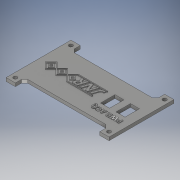
# Autodesk Inventor part: MapleMiniCase_TopCover
Saved by Autodesk Inventor 2018 (Build 220112000, 112)
## iProperties
Created: 2019-01-14
Part Number: MapleMiniCase_TopCover
Material: Generic
Document SubType Name: Modeling
Designer: tbrow
Density: 1 g/cm^3
Appearance: Default
Author: tbrow
## iProperties of the stored document MapleMiniCase_TopCover_3DPrint.ipt
Created: 2019-01-15
Part Number: MapleMiniCase_TopCover_3DPrint
Material: Generic
Document SubType Name: Modeling
Designer: tbrow
Density: 1 g/cm^3
Appearance: Default
Author: tbrow
Autodesk Inventor part; units mm, degrees
ref_plane "YZ Plane" through (0, 0, 0) normal (1, 0, 0) x (0, 1, 0)
ref_plane "XZ Plane" through (0, 0, 0) normal (0, 1, 0) x (-1, 0, 0)
ref_plane "XY Plane" through (0, 0, 0) normal (0, 0, 1) x (1, 0, 0)
sketch "Sketch1" plane through (0, 0, 0) normal (0, 1, 0) x (-1, 0, 0)
  line L0 (0, 0) -> (9.144, 0)
  line L1 (9.144, 0) -> (9.144, -9.144)
  line L2 (9.144, -9.144) -> (89.916, -9.144)
  line L3 (89.916, -9.144) -> (89.916, 0)
  line L4 (89.916, 0) -> (99.06, 0)
  line L5 (99.06, 0) -> (99.06, -58.6994)
  line L6 (99.06, -58.6994) -> (89.916, -58.6994)
  line L7 (89.916, -58.6994) -> (89.916, -49.5554)
  line L8 (89.916, -49.5554) -> (9.144, -49.5554)
  line L9 (9.144, -49.5554) -> (9.144, -58.6994)
  line L10 (9.144, -58.6994) -> (0, -58.6994)
  line L11 (0, -58.6994) -> (0, 0)
  dimension "d0" = 58.6994
  dimension "d1" = 9.144
  dimension "d2" = 9.144
  dimension "d3" = 9.144
  dimension "d4" = 9.144
  dimension "d5" = 9.144
  dimension "d7" = 9.144
  dimension "d16" = 99.06
  constraints: 24 end point, 8 perpendicular, 4 point on line, 2 horizontal
  measures "d0" distance of L4.end L5.end
  measures "d1" distance of L3.end L4.end
  measures "d2" distance of L2.end L3.end
  measures "d3" distance of L6.end L7.end
  measures "d4" distance of L0.start L0.end
  measures "d5" distance of L9.end L10.end
  measures "d7" distance of L5.end L6.end
  measures "d16" distance between parallel lines of L11 L5
extrude "Extrusion1" add sketch "Sketch1" along normal blind 3.175
sketch "Sketch2" plane through (0, 3.175, 0) normal (0, 1, 0) x (1, 0, 0)
  line L0 (-99.06, 0) -> (-89.916, 0) projected
  line L1 (-89.916, 58.6994) -> (-99.06, 58.6994) projected
  line L2 (-89.916, 49.5554) -> (-89.916, 58.6994) projected
  line L3 (-89.916, 0) -> (-89.916, 9.144) projected
  line L4 (-9.144, 0) -> (0, 0) projected
  line L5 (-9.144, 9.144) -> (-9.144, 0) projected
  line L6 (-9.144, 58.6994) -> (-9.144, 49.5554) projected
  circle A0 centre (-94.488, 4.572) radius 1.8542
  circle A1 centre (-94.488, 54.102) radius 1.8542
  circle A2 centre (-4.572, 54.102) radius 1.8542
  circle A3 centre (-4.572, 4.572) radius 1.8542
  line L7 (-99.06, 58.6994) -> (-99.06, 0) projected
  line L8 (0, 58.6994) -> (-9.144, 58.6994) projected
  line L9 (0, 0) -> (0, 58.6994) projected
  dimension "d10" = 3.7084
  dimension "d11" = 3.7084
  dimension "d12" = 3.7084
  dimension "d13" = 3.7084
  dimension "d17" = 4.572
  dimension "d18" = 4.5974
  dimension "d19" = 4.572
  dimension "d20" = 4.572
  dimension "d21" = 4.5974
  dimension "d22" = 4.572
  dimension "d23" = 4.572
  dimension "d24" = 4.572
  constraints: 4 centre point
  measures "d10" diameter of A0
  measures "d11" diameter of A1
  measures "d12" diameter of A2
  measures "d13" diameter of A3
  measures "d17" distance from line of L2 A1.centre
  measures "d18" distance from line of L1 A1.centre
  measures "d19" distance from line of L7 A0.centre
  measures "d20" distance from line of L0 A0.centre
  measures "d21" distance from line of L8 A2.centre
  measures "d22" distance from line of L9 A2.centre
  measures "d23" distance from line of L9 A3.centre
  measures "d24" distance from line of L4 A3.centre
extrude "Extrusion2" cut sketch "Sketch2" against normal blind 25.4
sketch "Sketch3" plane through (0, 3.175, 0) normal (0, 1, 0) x (1, 0, 0)
  line L0 (-33.274, 36.4617) -> (-24.384, 36.4617)
  line L1 (-24.384, 36.4617) -> (-24.384, 22.2377)
  line L2 (-24.384, 22.2377) -> (-33.274, 22.2377)
  line L3 (-33.274, 22.2377) -> (-33.274, 36.4617)
  line L4 (-18.034, 36.4617) -> (-9.144, 36.4617)
  line L5 (-9.144, 36.4617) -> (-9.144, 22.2377)
  line L6 (-9.144, 22.2377) -> (-18.034, 22.2377)
  line L7 (-18.034, 22.2377) -> (-18.034, 36.4617)
  line L8 (0, 0) -> (0, 58.6994) projected
  line L9 (0, 29.3497) -> (-99.06, 29.3497) construction
  line L10 (-99.06, 58.6994) -> (-99.06, 0) projected
  line L11 (-33.274, 29.3497) -> (-24.384, 29.3497) construction
  line L12 (-9.144, 29.3497) -> (-18.034, 29.3497) construction
  dimension "d25" = 14.224
  dimension "d26" = 8.89
  dimension "d27" = 8.89
  dimension "d28" = 6.35
  dimension "d32" = 9.144
  constraints: 22 end point, 6 midpoint, 4 parallel, 2 horizontal, 2 perpendicular, 2 point on line, 1 collinear
  measures "d25" distance of L2.end L0.start
  measures "d26" distance of L0.start L0.end
  measures "d27" distance of L4.start L4.end
  measures "d28" distance between parallel lines of L7 L1
  measures "d32" distance between parallel lines of L8 L5
extrude "Extrusion3" cut sketch "Sketch3" against normal blind 25.4
sketch "Sketch5" plane through (0, 3.175, 0) normal (0, 1, 0) x (1, 0, 0)
  line L0 (-7.013237, 13.615585) -> (-20.164763, 13.615585) construction
  line L1 (-20.164763, 13.615585) -> (-20.164763, 19.339606) construction
  line L2 (-20.164763, 19.339606) -> (-7.013237, 19.339606) construction
  line L3 (-7.013237, 19.339606) -> (-7.013237, 13.615585) construction
  line L4 (-24.384, 22.2377) -> (-33.274, 22.2377)
  line L5 (-13.589, 13.615585) -> (-13.589, 11.612972) construction
  line L6 (-18.034, 22.2377) -> (-9.144, 22.2377)
  line L7 (-13.589, 22.2377) -> (-13.589, 19.08791) construction
  line L8 (-10.651094, 22.2377) -> (-10.651094, 9.144) construction
  line L9 (-89.916, 9.144) -> (-9.144, 9.144)
  line L10 (-10.651094, 15.69085) -> (6.071001, 15.69085) construction
  line L11 (-24.334109, 13.528015) -> (-33.323891, 13.528015) construction
  line L12 (-33.323891, 13.528015) -> (-33.323891, 20.193969) construction
  line L13 (-33.323891, 20.193969) -> (-24.334109, 20.193969) construction
  line L14 (-24.334109, 20.193969) -> (-24.334109, 13.528015) construction
  line L15 (-33.274, 22.2377) -> (-33.274, 36.4617)
  line L16 (-28.829, 13.528015) -> (-28.829, 6.185177) construction
  line L17 (-33.274, 22.2377) -> (-24.384, 22.2377)
  line L18 (-28.829, 22.2377) -> (-28.829, 19.08791) construction
  line L19 (-13.589, 17.466453) -> (-13.589, 15.05585) construction
  line L20 (-28.829, 17.466453) -> (-28.829, 17.425462) construction
  spline S0 degree 2 poles (-10.100359, 15.016805) (-10.100359, 15.326586) (-9.902243, 15.888514) (-9.718536, 16.075824) knots 0 0 0 1 2 2 2
  spline S1 degree 2 poles (-9.718536, 16.075824) (-9.606871, 16.194694) (-9.333111, 16.389207) (-9.171016, 16.457647) knots 0 0 0 1 2 2 2
  spline S2 degree 2 poles (-9.171016, 16.457647) (-9.005319, 16.526087) (-8.619893, 16.605334) (-8.382154, 16.605334) knots 0 0 0 1 2 2 2
  line L21 (-8.382154, 16.605334) -> (-7.798613, 16.605334)
  line L22 (-7.798613, 16.605334) -> (-7.798613, 18.060585)
  line L23 (-7.798613, 18.060585) -> (-6.68196, 18.060585)
  line L24 (-6.68196, 18.060585) -> (-6.68196, 13.615585)
  line L25 (-6.68196, 13.615585) -> (-8.407369, 13.615585)
  spline S3 degree 2 poles (-8.407369, 13.615585) (-8.789192, 13.615585) (-9.347519, 13.756067) (-9.574452, 13.907356) knots 0 0 0 1 2 2 2
  spline S4 degree 2 poles (-9.574452, 13.907356) (-9.826599, 14.076655) (-10.100359, 14.631379) (-10.100359, 15.016805) knots 0 0 0 1 2 2 2
  spline S5 degree 2 poles (-8.954889, 15.045621) (-8.954889, 14.85471) (-8.774784, 14.584552) (-8.652312, 14.534122) knots 0 0 0 1 2 2 2
  spline S6 degree 2 poles (-8.652312, 14.534122) (-8.49382, 14.465682) (-8.205651, 14.44407) (-7.957106, 14.44407) knots 0 0 0 1 2 2 2
  line L26 (-7.957106, 14.44407) -> (-7.798613, 14.44407)
  line L27 (-7.798613, 14.44407) -> (-7.798613, 15.776849)
  line L28 (-7.798613, 15.776849) -> (-7.877859, 15.776849)
  spline S7 degree 2 poles (-7.877859, 15.776849) (-8.03275, 15.776849) (-8.313714, 15.769645) (-8.418175, 15.751634) knots 0 0 0 1 2 2 2
  spline S8 degree 2 poles (-8.418175, 15.751634) (-8.508228, 15.737226) (-8.706344, 15.650775) (-8.760376, 15.596744) knots 0 0 0 1 2 2 2
  spline S9 degree 2 poles (-8.760376, 15.596744) (-8.875643, 15.488681) (-8.954889, 15.247339) (-8.954889, 15.045621) knots 0 0 0 1 2 2 2
  line L29 (-16.429261, 13.615585) -> (-15.305404, 18.060585)
  line L30 (-15.305404, 18.060585) -> (-14.080688, 18.060585)
  line L31 (-14.080688, 18.060585) -> (-13.36747, 15.312177)
  line L32 (-13.36747, 15.312177) -> (-12.679468, 18.060585)
  line L33 (-12.679468, 18.060585) -> (-11.451149, 18.060585)
  line L34 (-11.451149, 18.060585) -> (-10.327292, 13.615585)
  line L35 (-10.327292, 13.615585) -> (-11.487171, 13.615585)
  line L36 (-11.487171, 13.615585) -> (-12.099529, 16.590925)
  line L37 (-12.099529, 16.590925) -> (-12.841563, 13.615585)
  line L38 (-12.841563, 13.615585) -> (-13.951012, 13.615585)
  line L39 (-13.951012, 13.615585) -> (-14.657025, 16.594527)
  line L40 (-14.657025, 16.594527) -> (-15.2982, 13.615585)
  line L41 (-15.2982, 13.615585) -> (-16.429261, 13.615585)
  line L42 (-21.086786, 18.060585) -> (-19.728791, 18.060585)
  line L43 (-19.728791, 18.060585) -> (-18.493269, 16.428831)
  line L44 (-18.493269, 16.428831) -> (-18.089833, 16.428831)
  line L45 (-18.089833, 16.428831) -> (-18.089833, 18.060585)
  line L46 (-18.089833, 18.060585) -> (-16.980384, 18.060585)
  line L47 (-16.980384, 18.060585) -> (-16.980384, 13.615585)
  line L48 (-16.980384, 13.615585) -> (-18.767029, 13.615585)
  spline S10 degree 2 poles (-18.767029, 13.615585) (-19.138046, 13.615585) (-19.685566, 13.70924) (-19.919703, 13.853324) knots 0 0 0 1 2 2 2
  spline S11 degree 2 poles (-19.919703, 13.853324) (-20.157442, 14.004613) (-20.438406, 14.476489) (-20.438406, 14.836699) knots 0 0 0 1 2 2 2
  spline S12 degree 2 poles (-20.438406, 14.836699) (-20.438406, 15.344596) (-19.977337, 15.982169) (-19.591911, 16.169479) knots 0 0 0 1 2 2 2
  line L49 (-19.591911, 16.169479) -> (-21.086786, 18.060585)
  spline S13 degree 2 poles (-19.292936, 14.977181) (-19.292936, 14.807882) (-19.16326, 14.566541) (-19.015574, 14.501703) knots 0 0 0 1 2 2 2
  spline S14 degree 2 poles (-19.015574, 14.501703) (-18.911113, 14.458478) (-18.655363, 14.433263) (-18.464452, 14.433263) knots 0 0 0 1 2 2 2
  line L50 (-18.464452, 14.433263) -> (-18.089833, 14.433263)
  line L51 (-18.089833, 14.433263) -> (-18.089833, 15.629163)
  line L52 (-18.089833, 15.629163) -> (-18.41042, 15.629163)
  spline S15 degree 2 poles (-18.41042, 15.629163) (-18.640955, 15.629163) (-18.968747, 15.571529) (-19.080412, 15.481476) knots 0 0 0 1 2 2 2
  spline S16 degree 2 poles (-19.080412, 15.481476) (-19.188475, 15.395026) (-19.292936, 15.164491) (-19.292936, 14.977181) knots 0 0 0 1 2 2 2
  line L53 (-22.323595, 18.066669) -> (-23.825673, 13.621669)
  line L54 (-23.825673, 13.621669) -> (-25.043186, 13.621669)
  line L55 (-25.043186, 13.621669) -> (-26.545264, 18.066669)
  line L56 (-26.545264, 18.066669) -> (-25.396192, 18.066669)
  line L57 (-25.396192, 18.066669) -> (-25.11883, 17.158938)
  line L58 (-25.11883, 17.158938) -> (-23.721212, 17.158938)
  line L59 (-23.721212, 17.158938) -> (-23.440248, 18.066669)
  line L60 (-23.440248, 18.066669) -> (-22.323595, 18.066669)
  line L61 (-24.873887, 16.352066) -> (-24.420021, 14.882407)
  line L62 (-24.420021, 14.882407) -> (-23.962554, 16.352066)
  line L63 (-23.962554, 16.352066) -> (-24.873887, 16.352066)
  spline S17 degree 2 poles (-28.904644, 18.15312) (-27.903259, 18.15312) (-26.728972, 16.942812) (-26.728972, 15.847771) knots 0 0 0 1 2 2 2
  spline S18 degree 2 poles (-26.728972, 15.847771) (-26.728972, 14.792354) (-27.906861, 13.535219) (-28.908246, 13.535219) knots 0 0 0 1 2 2 2
  spline S19 degree 2 poles (-28.908246, 13.535219) (-29.1712, 13.535219) (-29.596249, 13.596455) (-29.790763, 13.646884) knots 0 0 0 1 2 2 2
  spline S20 degree 2 poles (-29.790763, 13.646884) (-29.942051, 13.693712) (-30.29866, 13.848602) (-30.410325, 13.906236) knots 0 0 0 1 2 2 2
  line L64 (-30.410325, 13.906236) -> (-30.410325, 14.965255)
  line L65 (-30.410325, 14.965255) -> (-30.29866, 14.965255)
  spline S21 degree 2 poles (-30.29866, 14.965255) (-30.215811, 14.893213) (-29.970868, 14.691495) (-29.815977, 14.59784) knots 0 0 0 1 2 2 2
  spline S22 degree 2 poles (-29.815977, 14.59784) (-29.661087, 14.500583) (-29.29007, 14.367306) (-29.08475, 14.367306) knots 0 0 0 1 2 2 2
  spline S23 degree 2 poles (-29.08475, 14.367306) (-28.843408, 14.367306) (-28.443575, 14.518594) (-28.259867, 14.709506) knots 0 0 0 1 2 2 2
  spline S24 degree 2 poles (-28.259867, 14.709506) (-28.09417, 14.878805) (-27.881646, 15.458744) (-27.881646, 15.851374) knots 0 0 0 1 2 2 2
  spline S25 degree 2 poles (-27.881646, 15.851374) (-27.881646, 16.265616) (-28.101374, 16.831147) (-28.28148, 17.004048) knots 0 0 0 1 2 2 2
  spline S26 degree 2 poles (-28.28148, 17.004048) (-28.454381, 17.173347) (-28.87943, 17.321033) (-29.091954, 17.321033) knots 0 0 0 1 2 2 2
  spline S27 degree 2 poles (-29.091954, 17.321033) (-29.311682, 17.321033) (-29.711516, 17.173347) (-29.848396, 17.083294) knots 0 0 0 1 2 2 2
  spline S28 degree 2 poles (-29.848396, 17.083294) (-29.999685, 16.993242) (-30.226618, 16.80233) (-30.309466, 16.726686) knots 0 0 0 1 2 2 2
  line L66 (-30.309466, 16.726686) -> (-30.410325, 16.726686)
  line L67 (-30.410325, 16.726686) -> (-30.410325, 17.771297)
  spline S29 degree 2 poles (-30.410325, 17.771297) (-30.287853, 17.82893) (-29.967266, 17.973015) (-29.794365, 18.023444) knots 0 0 0 1 2 2 2
  spline S30 degree 2 poles (-29.794365, 18.023444) (-29.585443, 18.088282) (-29.22163, 18.15312) (-28.904644, 18.15312) knots 0 0 0 1 2 2 2
  spline S31 degree 2 poles (-35.107473, 19.240956) (-34.927367, 19.284182) (-34.567156, 19.327407) (-34.181731, 19.327407) knots 0 0 0 1 2 2 2
  spline S32 degree 2 poles (-34.181731, 19.327407) (-33.832327, 19.327407) (-33.338838, 19.150904) (-33.173141, 18.988809) knots 0 0 0 1 2 2 2
  spline S33 degree 2 poles (-33.173141, 18.988809) (-33.011046, 18.830316) (-32.845349, 18.398063) (-32.834543, 18.145916) knots 0 0 0 1 2 2 2
  spline S34 degree 2 poles (-32.834543, 18.145916) (-31.894393, 18.10269) (-30.810159, 16.881576) (-30.810159, 15.844169) knots 0 0 0 1 2 2 2
  spline S35 degree 2 poles (-30.810159, 15.844169) (-30.810159, 14.774344) (-31.955629, 13.528015) (-32.960617, 13.528015) knots 0 0 0 1 2 2 2
  spline S36 degree 2 poles (-32.960617, 13.528015) (-33.962002, 13.528015) (-35.114677, 14.767139) (-35.114677, 15.844169) knots 0 0 0 1 2 2 2
  spline S37 degree 2 poles (-35.114677, 15.844169) (-35.114677, 16.629429) (-34.462695, 17.753286) (-33.864746, 17.991025) knots 0 0 0 1 2 2 2
  spline S38 degree 2 poles (-33.864746, 17.991025) (-33.87195, 18.318817) (-34.149312, 18.567362) (-34.495114, 18.567362) knots 0 0 0 1 2 2 2
  spline S39 degree 2 poles (-34.495114, 18.567362) (-34.631994, 18.567362) (-34.930969, 18.488116) (-34.995807, 18.452095) knots 0 0 0 1 2 2 2
  line L68 (-34.995807, 18.452095) -> (-35.107473, 18.452095)
  line L69 (-35.107473, 18.452095) -> (-35.107473, 19.240956)
  spline S40 degree 2 poles (-33.663028, 16.968027) (-33.807112, 16.773513) (-33.962002, 16.258412) (-33.962002, 15.840567) knots 0 0 0 1 2 2 2
  spline S41 degree 2 poles (-33.962002, 15.840567) (-33.962002, 15.444336) (-33.799908, 14.886009) (-33.659426, 14.705904) knots 0 0 0 1 2 2 2
  spline S42 degree 2 poles (-33.659426, 14.705904) (-33.518943, 14.525798) (-33.158733, 14.367306) (-32.964219, 14.367306) knots 0 0 0 1 2 2 2
  spline S43 degree 2 poles (-32.964219, 14.367306) (-32.758899, 14.367306) (-32.423903, 14.514992) (-32.269012, 14.702301) knots 0 0 0 1 2 2 2
  spline S44 degree 2 poles (-32.269012, 14.702301) (-32.132132, 14.875203) (-31.962833, 15.447938) (-31.962833, 15.844169) knots 0 0 0 1 2 2 2
  spline S45 degree 2 poles (-31.962833, 15.844169) (-31.962833, 16.251207) (-32.124928, 16.791524) (-32.26541, 16.975231) knots 0 0 0 1 2 2 2
  spline S46 degree 2 poles (-32.26541, 16.975231) (-32.405892, 17.158938) (-32.769705, 17.317431) (-32.964219, 17.317431) knots 0 0 0 1 2 2 2
  spline S47 degree 2 poles (-32.964219, 17.317431) (-33.162335, 17.317431) (-33.52975, 17.148132) (-33.663028, 16.968027) knots 0 0 0 1 2 2 2
  point P0 (0, 0)
  dimension "d34" = 270
  dimension "d35" = 270
  constraints: 16 end point, 7 vertical, 5 midpoint, 4 collinear, 2 point on line, 1 horizontal, 4 other
emboss "Emboss1" sketch "Sketch5" operation add depth 0.508 direction (0, -1, 0)
sketch "Sketch6" plane through (0, 3.175, 0) normal (0, 1, 0) x (1, 0, 0)
  line L0 (-40.37026, 23.424425) -> (-65.03083, 23.424425)
  line L1 (-67.69783, 24.262625) -> (-40.37026, 24.262625)
  line L2 (-40.37026, 24.262625) -> (-40.37026, 23.424425)
  line L3 (-56.772203, 24.897625) -> (-54.733411, 24.897625) construction
  line L4 (-37.83026, 42.201375) -> (-37.83026, 16.483875) construction
  line L5 (-37.217834, 34.422627) -> (-67.697834, 34.422627)
  line L6 (-67.697834, 34.422627) -> (-67.697834, 35.248127) construction
  line L7 (-67.697834, 35.248127) -> (-37.217834, 35.248127)
  line L8 (-37.217834, 35.248127) -> (-37.217834, 34.422627)
  line L9 (-51.606785, 33.787627) -> (-53.753641, 33.787627) construction
  line L10 (-64.81776, 29.342625) -> (-67.96085, 26.199535)
  line L11 (-67.96085, 26.199535) -> (-71.103939, 29.342625)
  line L12 (-71.103939, 29.342625) -> (-67.96085, 32.485715)
  line L13 (-67.96085, 32.485715) -> (-64.81776, 29.342625)
  line L14 (-67.96085, 26.199535) -> (-67.96085, 32.485715) construction
  line L15 (-69.487493, 29.342625) -> (-67.96085, 27.815981)
  line L16 (-67.96085, 27.815981) -> (-66.434206, 29.342625)
  line L17 (-66.434206, 29.342625) -> (-67.96085, 30.869268)
  line L18 (-67.96085, 30.869268) -> (-69.487493, 29.342625)
  line L19 (-65.03083, 23.424425) -> (-67.96085, 23.424425)
  line L20 (-67.697834, 35.248127) -> (-67.96086, 35.248127)
  line L21 (-73.226843, 28.690418) -> (-73.226843, 24.437088) construction
  line L22 (-81.635926, 29.342625) -> (-78.492837, 26.199535)
  line L23 (-78.492837, 27.815981) -> (-80.01948, 29.342625)
  line L24 (-76.966193, 29.342625) -> (-78.492837, 27.815981)
  line L25 (-78.492837, 26.199535) -> (-75.349747, 29.342625)
  line L26 (-75.349747, 29.342625) -> (-78.492837, 32.485715)
  line L27 (-78.492837, 30.869268) -> (-76.966193, 29.342625)
  line L28 (-80.01948, 29.342625) -> (-78.492837, 30.869268)
  line L29 (-78.492837, 32.485715) -> (-81.635926, 29.342625)
  line L30 (-83.758819, 28.690412) -> (-83.758819, 23.231829) construction
  line L31 (-85.881712, 29.342625) -> (-89.024802, 26.199535)
  line L32 (-89.024802, 26.199535) -> (-92.167891, 29.342625)
  line L33 (-90.551445, 29.342625) -> (-89.024802, 27.815981)
  line L34 (-89.024802, 27.815981) -> (-87.498158, 29.342625)
  line L35 (-92.167891, 29.342625) -> (-89.024802, 32.485715)
  line L36 (-89.024802, 30.869268) -> (-90.551445, 29.342625)
  line L37 (-87.498158, 29.342625) -> (-89.024802, 30.869268)
  line L38 (-89.024802, 32.485715) -> (-85.881712, 29.342625)
  line L39 (-88.996085, 24.554373) -> (-93.784337, 29.342625)
  line L40 (-89.035539, 23.413693) -> (-94.958121, 29.336275)
  line L41 (-88.996084, 34.130878) -> (-93.784337, 29.342625)
  line L42 (-89.035538, 35.258857) -> (-94.958121, 29.336275)
  line L43 (-78.492834, 35.248127) -> (-83.758821, 29.98214)
  line L44 (-84.207832, 29.342626) -> (-88.996085, 24.554373)
  line L45 (-78.49283, 34.159599) -> (-83.309805, 29.342625)
  line L46 (-83.758819, 28.690412) -> (-89.035539, 23.413693)
  line L47 (-78.49283, 24.52565) -> (-83.309805, 29.342625)
  line L48 (-83.758821, 29.98214) -> (-89.035538, 35.258857)
  line L49 (-78.492834, 23.424427) -> (-83.758819, 28.690412)
  line L50 (-84.207832, 29.342626) -> (-88.996084, 34.130878)
  line L51 (-67.96085, 23.424425) -> (-73.226843, 28.690418)
  line L52 (-73.675856, 29.342625) -> (-78.49283, 34.159599)
  line L53 (-67.69783, 24.262625) -> (-72.777833, 29.342628)
  line L54 (-73.226847, 29.98214) -> (-78.492834, 35.248127)
  line L55 (-67.697834, 34.422627) -> (-72.777833, 29.342628)
  line L56 (-73.226843, 28.690418) -> (-78.492834, 23.424427)
  line L57 (-67.96086, 35.248127) -> (-73.226847, 29.98214)
  line L58 (-73.675856, 29.342625) -> (-78.49283, 24.52565)
  line L59 (-89.916, 58.6994) -> (-99.06, 58.6994)
  line L60 (-33.274, 22.2377) -> (-33.274, 36.4617)
  line L61 (-44.286596, 24.262625) -> (-44.286596, 34.422627) construction
  line L62 (-44.286596, 29.342626) -> (-40.109376, 29.342626) construction
  line L63 (-33.274, 29.3497) -> (-111.455813, 29.3497) construction
  line L64 (-39.258262, 25.002588) -> (-65.70747, 25.002588) construction
  line L65 (-65.70747, 25.002588) -> (-65.70747, 34.711002) construction
  line L66 (-65.70747, 34.711002) -> (-39.258262, 34.711002) construction
  line L67 (-39.258262, 34.711002) -> (-39.258262, 25.002588) construction
  line L68 (-89.916, 9.144) -> (-9.144, 9.144)
  line L69 (-53.541106, 25.002588) -> (-53.541106, 24.262625) construction
  spline S0 degree 2 poles (-45.179431, 30.362977) (-44.577418, 32.152523) (-42.276574, 34.049276) (-40.709691, 34.049276) knots 0 0 0 1 2 2 2
  spline S1 degree 2 poles (-40.709691, 34.049276) (-40.008717, 34.049276) (-39.489171, 33.801873) knots 0 0 0 1 1 1
  line L70 (-39.489171, 33.801873) -> (-40.132418, 31.92986)
  spline S2 degree 2 poles (-40.132418, 31.92986) (-40.511768, 32.317458) (-41.155015, 32.317458) knots 0 0 0 1 1 1
  spline S3 degree 2 poles (-41.155015, 32.317458) (-42.523976, 32.317458) (-43.216704, 30.28051) knots 0 0 0 1 1 1
  line L71 (-43.216704, 30.28051) -> (-45.006249, 25.002588)
  line L72 (-45.006249, 25.002588) -> (-47.001963, 25.002588)
  line L73 (-47.001963, 25.002588) -> (-45.179431, 30.362977)
  line L74 (-53.929236, 33.892587) -> (-51.908781, 33.892587)
  line L75 (-51.908781, 33.892587) -> (-50.143976, 28.301289)
  spline S4 degree 2 poles (-50.143976, 28.301289) (-49.987288, 27.81473) (-49.946054, 27.567328) knots 0 0 0 1 1 1
  line L76 (-49.946054, 27.567328) -> (-49.921314, 27.567328)
  spline S5 degree 2 poles (-49.921314, 27.567328) (-49.814106, 28.037393) (-49.484236, 29.002263) knots 0 0 0 1 1 1
  line L77 (-49.484236, 29.002263) -> (-47.826639, 33.892587)
  line L78 (-47.826639, 33.892587) -> (-45.929885, 33.892587)
  line L79 (-45.929885, 33.892587) -> (-48.956444, 25.002588)
  line L80 (-48.956444, 25.002588) -> (-51.108846, 25.002588)
  line L81 (-51.108846, 25.002588) -> (-52.799431, 30.412458)
  spline S6 degree 2 poles (-52.799431, 30.412458) (-52.914885, 30.783562) (-52.997353, 31.138172) knots 0 0 0 1 1 1
  line L82 (-52.997353, 31.138172) -> (-53.022093, 31.138172)
  spline S7 degree 2 poles (-53.022093, 31.138172) (-53.07982, 30.833042) (-53.393197, 29.917652) knots 0 0 0 1 1 1
  line L83 (-53.393197, 29.917652) -> (-55.059041, 25.002588)
  line L84 (-55.059041, 25.002588) -> (-56.955794, 25.002588)
  line L85 (-56.955794, 25.002588) -> (-53.929236, 33.892587)
  line L86 (-63.429496, 33.892587) -> (-61.128652, 33.892587)
  line L87 (-61.128652, 33.892587) -> (-60.526639, 31.608237)
  spline S8 degree 2 poles (-60.526639, 31.608237) (-60.460665, 31.344341) (-60.312223, 30.932003) (-60.114301, 30.643367) (-59.850405, 30.486678) (-59.668976, 30.486678) knots 0 0 0 1 2 3 4 4 4
  line L88 (-59.668976, 30.486678) -> (-59.132937, 30.486678)
  line L89 (-59.132937, 30.486678) -> (-57.970145, 33.892587)
  line L90 (-57.970145, 33.892587) -> (-55.966184, 33.892587)
  line L91 (-55.966184, 33.892587) -> (-58.992742, 25.002588)
  line L92 (-58.992742, 25.002588) -> (-62.167742, 25.002588)
  spline S9 degree 2 poles (-62.167742, 25.002588) (-65.40047, 25.002588) (-64.584041, 27.418886) knots 0 0 0 1 1 1
  spline S10 degree 2 poles (-64.584041, 27.418886) (-64.419106, 27.880704) (-63.866574, 28.672393) (-63.132613, 29.307393) (-62.241963, 29.760964) (-61.747158, 29.892912) knots 0 0 0 1 2 3 4 4 4
  line L93 (-61.747158, 29.892912) -> (-61.738911, 29.917652)
  spline S11 degree 2 poles (-61.738911, 29.917652) (-61.912093, 29.983626) (-62.192483, 30.255769) (-62.406898, 30.626873) (-62.58008, 31.055704) (-62.646054, 31.261873) knots 0 0 0 1 2 3 4 4 4
  line L94 (-62.646054, 31.261873) -> (-63.429496, 33.892587)
  line L95 (-60.485405, 26.503497) -> (-59.644236, 28.977523)
  line L96 (-59.644236, 28.977523) -> (-60.510145, 28.977523)
  spline S12 degree 2 poles (-60.510145, 28.977523) (-61.153392, 28.977523) (-61.672937, 28.606419) knots 0 0 0 1 1 1
  spline S13 degree 2 poles (-61.672937, 28.606419) (-62.200729, 28.227068) (-62.390405, 27.666289) knots 0 0 0 1 1 1
  spline S14 degree 2 poles (-62.390405, 27.666289) (-62.786249, 26.503497) (-61.392548, 26.503497) knots 0 0 0 1 1 1
  line L97 (-61.392548, 26.503497) -> (-60.485405, 26.503497)
  point P0 (0, 0)
  dimension "d39" = 0.8382
  dimension "d40" = 0.635
  dimension "d41" = 2.54
  dimension "d42" = 30.48
  dimension "d43" = 0.635
  dimension "d44" = 0.8255
  dimension "d45" = 45
  dimension "d46" = 10.16
  dimension "d47" = 5.08
  dimension "d48" = 4.445
  dimension "d49" = 4.445
  dimension "d50" = 26.9875
  dimension "d51" = 1.143
  dimension "d52" = 0.83448
  dimension "d53" = 1.143
  dimension "d54" = 0.8255
  dimension "d55" = 1.143
  dimension "d56" = 0
  dimension "d59" = 270
  constraints: 126 end point, 35 parallel, 16 symmetric about line, 5 perpendicular, 4 point on line, 2 horizontal, 2 midpoint, 5 other
  measures "d39" distance of L1.end L0.start
  measures "d40" distance between parallel lines of L1 L3
  measures "d41" distance between parallel lines of L4 L2
  measures "d42" distance of L20.start L7.end
  measures "d43" distance between parallel lines of L5 L9
  measures "d44" distance of L55.start L20.start
  measures "d45" angle of L5 L13
  measures "d46" distance between parallel lines of L5 L1
  measures "d47" distance from line of L1 L13.end
  measures "d48" distance of L13.end L14.start
  measures "d49" distance of L12.end L13.end
  measures "d50" distance from line of L4 L13.end
  measures "d51" distance between parallel lines of L11 L15
  measures "d52" distance between parallel lines of L40 L39
  measures "d53" distance between parallel lines of L39 L32
  measures "d54" distance between parallel lines of L42 L41
  measures "d55" distance between parallel lines of L35 L41
  measures "d56" horizontal distance of L19.end L14.start
emboss "Emboss2" sketch "Sketch6" operation add depth 0.762 direction (0, -1, 0)
sketch "Sketch7" plane through (0, 3.175, 0) normal (0, 1, 0) x (1, 0, 0)
  line L0 (-40.132418, 31.92986) -> (-39.489171, 33.801873)
  line L1 (-40.132418, 31.92986) -> (-44.202912, 20.083677)
  line L2 (-39.489171, 33.801873) -> (-37.418018, 39.82946)
  line L3 (-37.418018, 39.82946) -> (-35.999557, 37.571819)
  line L4 (-35.999557, 37.571819) -> (-36.707895, 19.785194)
  line L5 (-36.707895, 19.785194) -> (-44.202912, 20.083677)
  point P0 (0, 0)
  constraints: 10 end point, 2 collinear, 1 perpendicular
extrude "Extrusion4" cut sketch "Sketch7" along normal blind 25.4
chamfer "Chamfer1" distance 3.175 angle 45 4 edges at (-89.916, 1.5875, -49.5554) (-9.144, 1.5875, -49.5554) (-9.144, 1.5875, -9.144) (-89.916, 1.5875, -9.144)
move faces "Move1" translate (0, 0, 2.667) faces at (-37.126333, 1.058333, -9.144) (-89.916, 1.058333, -3.979333) (-94.562661, 1.058333, -6.424696) (-92.964, 1.058333, 0) (-2.723813, 1.058333, -4.422799) (-3.048, 1.058333, 0) (-11.260667, 1.058333, -8.085667) (-9.144, 1.058333, -1.989667) (-88.857667, 1.058333, -7.027333)
move faces "Move2" translate (0, 0, -2.667) faces at (-61.933667, 1.058333, -49.5554) (-92.639813, 1.058333, -53.952799) (-96.012, 1.058333, -58.6994) (-11.260667, 1.058333, -50.613733) (-9.144, 1.058333, -54.720067) (-6.096, 1.058333, -58.6994) (-2.723813, 1.058333, -53.952799) (-88.857667, 1.058333, -51.672067) (-89.916, 1.058333, -56.709733)
move faces "Move3" translate (-2.54, 0, 0) faces at (-93.005673, 2.116667, -55.655104) (-96.012, 1.058333, -61.3664) (-88.857667, 1.058333, -54.339067) (-89.916, 2.116667, -57.387067) (-94.413339, 1.058333, -3.757696) (-89.916, 2.116667, -1.312333) (-96.012, 2.116667, 2.667) (-88.857667, 1.058333, -4.360333) (-99.06, 1.058333, -18.677467)
equation "\"d2\" = d1"
equation "\"d3\" = d1"
equation "\"d4\" = d1"
equation "\"d5\" = d1"
equation "\"d7\" = d1"
equation "\"d19\" = d17"
equation "\"d20\" = d17"
equation "\"d22\" = d17"
equation "\"d23\" = d17"
equation "\"d24\" = d17"
body "Solid1"
